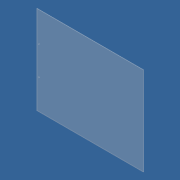
# Autodesk Inventor part: GE-12055
Saved by Autodesk Inventor 2012 (Build 160160000, 160)
## iProperties
Created: 2011-08-31
Part Number: GE-12055
Document SubType Name: Modeling
Designer: mcyr
Density: 1 g/cm^3
Description: Glass, Corner Driver Station
Material: Default
Title: Glass, Corner Driver Station
Author: mcyr
Autodesk Inventor part; units mm, degrees
ref_plane "YZ Plane" through (0, 0, 0) normal (1, 0, 0) x (0, 1, 0)
ref_plane "XZ Plane" through (0, 0, 0) normal (0, 1, 0) x (-1, 0, 0)
ref_plane "XY Plane" through (0, 0, 0) normal (0, 0, 1) x (1, 0, 0)
sketch "Sketch1" plane through (0, 0, 0) normal (0, 0, 1) x (1, 0, 0)
  line L0 (0, 0) -> (1270, 0)
  line L1 (1270, 0) -> (1270, 1054.1)
  line L2 (1270, 1054.1) -> (0, 1054.1)
  line L3 (0, 1054.1) -> (0, 0)
  dimension "d0" = 1054.1
  dimension "d1" = 1270
  constraints: 8 end point, 2 parallel, 1 horizontal, 1 perpendicular
  measures "d0" distance of L2.end L0.start
  measures "d1" distance of L0.start L0.end
extrude "Extrusion1" add sketch "Sketch1" along normal blind 6.35
hole "Hole1" at (25.4, 698.5, 6.35) direction (0, 0, -1) diameter 12.7 depth 25.4 tip angle 118
pattern_linear "Rectangular Pattern1" count 2 spacing 342.9 along (0, -1, 0) of "Hole1"
body "Solid1"
